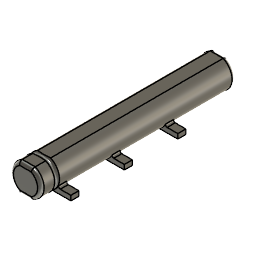
Shaft (Autodesk Fusion 360 design; units mm, degrees)
part number: 2026-05-27-20-57-14-897
part number: 2026-05-27-22-33-04-943
Autodesk Fusion 360 part; units mm, degrees
sketch "The front face" plane through (0, 0, 0) normal (0, 1, 0) x (1, 0, 0)
  circle A0 centre (0, 0) radius 4.75
  line L0 (-2, -4.3084) -> (2, -4.3084)
  line L1 (-2, 4.3084) -> (2, 4.3084)
  line L2 (0, -4.75) -> (0, 4.75) construction
  circle A1 centre (0, 0) radius 4
  dimension "d1" = 9.5
  dimension "d2" = 4
  dimension "d3" = 4
  dimension "d33" = 8
  constraint coincident A0.centre A1.centre
  constraint horizontal L0
  constraint coincident A0 L0.start
  constraint coincident A0 L0.end
  constraint horizontal L1
  constraint coincident A0 L1.start
  constraint coincident A0 L1.end
  constraint coincident A0 L2.start
  constraint coincident A0 L2.end
  constraint perpendicular L1 L2
  constraint concentric A0 A1
  measures "d1" diameter of A0
  measures "d2" distance of L0.start L0.end
  measures "d3" distance of L1.start L1.end
  measures "d33" diameter of A1
sketch "The path" plane through (0, 0, 0) normal (1, 0, 0) x (0, 1, 0)
  line L0 (0, 0) -> (60, 0)
  dimension "d4" = 60
  constraint coincident L0.start origin
  constraint horizontal L0
  measures "d4" distance of L0.start L0.end
sweep "Sweep1" add profiles "The front face" path "The path" along L0 section 1 contours A0 L0 L1 | A1 makes body 1
sketch "The bottom details" plane through (0, 0, -4.3084) normal (0, 0, -1) x (1, 0, 0)
  line L0 (2, 0) -> (-2, 0)
  line L1 (-2, 0) -> (-2, -60)
  line L2 (-2, -60) -> (2, -60)
  line L3 (2, -60) -> (2, 0)
  line L4 (2, 0) -> (2, -4) construction
  line L5 (2, -4) -> (2, -6) construction
  line L6 (2, -6) -> (2, -8.5) construction
  line L7 (2, -8.5) -> (2, -22.5) construction
  line L8 (2, -22.5) -> (2, -25) construction
  line L9 (2, -25) -> (2, -39) construction
  line L10 (2, -39) -> (2, -41.5) construction
  line L11 (2, -41.5) -> (2, -60) construction
  line L12 (2, -6) -> (8, -6)
  line L13 (8, -6) -> (8, -8.5)
  line L14 (8, -8.5) -> (2, -8.5)
  line L15 (2, -8.5) -> (2, -6)
  line L16 (8, -6) -> (5, -6)
  line L17 (5, -6) -> (5, -8.5)
  line L18 (5, -8.5) -> (8, -8.5)
  line L19 (8, -8.5) -> (8, -6)
  line L20 (2, -22.5) -> (8, -22.5)
  line L21 (8, -22.5) -> (8, -25)
  line L22 (8, -25) -> (2, -25)
  line L23 (2, -25) -> (2, -22.5)
  line L24 (2, -22.5) -> (5, -22.5)
  line L25 (5, -22.5) -> (5, -25)
  line L26 (5, -25) -> (2, -25)
  line L27 (2, -25) -> (2, -22.5)
  line L28 (2, -39) -> (8, -39)
  line L29 (8, -39) -> (8, -41.5)
  line L30 (8, -41.5) -> (2, -41.5)
  line L31 (2, -41.5) -> (2, -39)
  line L32 (2, -39) -> (5, -39)
  line L33 (5, -39) -> (5, -41.5)
  line L34 (5, -41.5) -> (2, -41.5)
  line L35 (2, -41.5) -> (2, -39)
  line L36 (2, -6) -> (2, -5.75) construction
  line L37 (2, -4) -> (2, -4.25) construction
  dimension "d11" = 4
  dimension "d12" = 2
  dimension "d13" = 2.5
  dimension "d14" = 14
  dimension "d15" = 2.5
  dimension "d16" = 14
  dimension "d17" = 2.5
  dimension "d18" = 18.5
  dimension "d19" = 6
  dimension "d20" = 3
  dimension "d21" = 6
  dimension "d22" = 3
  dimension "d23" = 2.5
  dimension "d24" = 6
  dimension "d31" = 0.25
  dimension "d32" = 0.25
  constraint coincident L0.start L3.end
  constraint perpendicular L0 L4
  constraint parallel L3 L5
  constraint parallel L3 L6
  constraint parallel L3 L7
  constraint parallel L3 L8
  constraint parallel L3 L9
  constraint parallel L3 L10
  constraint parallel L3 L11
  constraint horizontal L12
  constraint vertical L13
  constraint horizontal L14
  constraint vertical L15
  constraint horizontal L16
  constraint vertical L17
  constraint horizontal L18
  constraint vertical L19
  constraint horizontal L20
  constraint vertical L21
  constraint horizontal L22
  constraint vertical L23
  constraint horizontal L24
  constraint vertical L25
  constraint horizontal L26
  constraint vertical L27
  constraint horizontal L28
  constraint vertical L29
  constraint horizontal L30
  constraint vertical L31
  constraint horizontal L32
  constraint vertical L33
  constraint horizontal L34
  constraint vertical L35
  constraint midpoint L30 L33.end
  constraint perpendicular L12 L36
  constraint parallel L5 L37
  measures "d11" distance of L0.start L4.end
  measures "d12" distance of L4.end L5.end
  measures "d13" distance of L5.end L6.end
  measures "d14" distance of L6.end L7.end
  measures "d15" distance of L7.end L8.end
  measures "d16" distance of L8.end L9.end
  measures "d17" distance of L9.end L10.end
  measures "d18" distance of L10.end L2.end
  measures "d19" distance of L5.end L12.end
  measures "d20" distance of L12.end L16.end
  measures "d21" distance of L7.end L20.end
  measures "d22" distance of L7.end L24.end
  measures "d23" distance of L7.end L8.end
  measures "d24" distance of L9.end L28.end
  measures "d31" distance of L5.end L36.end
  measures "d32" distance of L4.end L37.end
extrude "Extrude1" add sketch "The bottom details" against normal blind 1.5 contours L3 L12 L14 L15 L17 | L12 L13 L14 L16 L17 L18 L19 bodies 1
extrude "Extrude2" add sketch "The bottom details" against normal blind 1.5 contours L3 L20 L22 L23 L24 L25 L26 L27 | L20 L21 L22 L25 bodies 1
extrude "Extrude3" add sketch "The bottom details" against normal blind 1.5 contours L3 L28 L30 L31 L32 L33 L34 L35 | L28 L29 L30 L33 bodies 1
extrude "Extrude4" cut sketch "The front face" along normal blind 1.5 from surface at 4.25 contours A0 L0 L1 bodies 1
fillet "Fillet1" radius 0.75 1 edges at (-3.7293, 5.75, -1.4465) on bodies 1
fillet "Fillet2" radius 0.75 1 edges at (-3.7293, 4.25, -1.4465) on bodies 1
fillet "Fillet3" radius 0.5 3 edges at (3.8308, 7.25, -2.8084) (3.8308, 23.75, -2.8084) (3.8308, 40.25, -2.8084) on bodies 1
fillet "Fillet4" radius 1 8 edges at (4.75, 0, 0) (-4.75, 0, 0) (0, 0, 4.3084) (0, 0, -4.3084) (0, 60, 4.3084) (-4.75, 60, 0) (0, 60, -4.3084) (4.75, 60, 0) on bodies 1
copy_body "Body->Comp1" bodies 1 removing the originals makes body 2 in component "Shaft (1)"
component "Shaft (1)" placed x (1, 0, 0) y (0, 1, 0) z (0, 0, 1) at (0, 0, 0)
named bodies: "Shaft"
